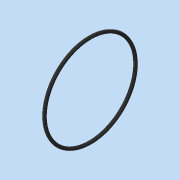
# Autodesk Inventor part: ORingA70_2.487ID_2.693OD_Compressed
Saved by Autodesk Inventor 2017 (Build 210142000, 142)
## iProperties
Created: 2016-11-26
Part Number: ORingA70_2.487ID_2.693OD_Compressed
Material: Rubber, Silicone
Document SubType Name: Modeling
Designer: techn
Density: 1.25 g/cm^3
Appearance: Rubber - Black
Author: techn
Autodesk Inventor part; units mm, degrees
ref_plane "YZ Plane" through (0, 0, 0) normal (1, 0, 0) x (0, 1, 0)
ref_plane "XZ Plane" through (0, 0, 0) normal (0, 1, 0) x (-1, 0, 0)
ref_plane "XY Plane" through (0, 0, 0) normal (0, 0, 1) x (1, 0, 0)
sketch "Sketch1" plane through (0, 0, 0) normal (0, 0, 1) x (1, 0, 0)
  line L0 (0, 0) -> (0, 32.7025)
  line L1 (0, 0) -> (0, 34.925)
  line L2 (0, 34.925) -> (0, 32.7025)
  ellipse E0 centre (0, 33.8137) end of major axis (0, 34.925) minor radius 1.2239
  line L3 (0, 0) -> (1.7541, 0)
  dimension "d0" = 32.7025
  dimension "d2" = 34.925
  constraints: 8 end point, 4 vertical, 1 horizontal, 1 midpoint, 1 vertical alignment, 2 other
  measures "d0" distance of L0.start L0.end
  measures "d2" distance of L0.start L1.end
revolve "Revolution1" add sketch "Sketch1" angle 360 about axis through (0, 0, 0) along (1, 0, 0)
body "Solid1"
